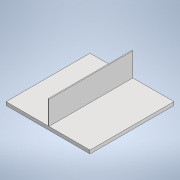
# Autodesk Inventor part: podłoga
Saved by Autodesk Inventor 2022.3 (Build 263350000, 350)
## iProperties
Created: 2023-01-17
Part Number: podłoga
Material: Generic
Document SubType Name: Modeling
Designer: komputer
Density: 1 g/cm^3
Appearance: Default
Author: komputer
Autodesk Inventor part; units mm, degrees
ref_plane "YZ Plane" through (0, 0, 0) normal (1, 0, 0) x (0, 1, 0)
ref_plane "XZ Plane" through (0, 0, 0) normal (0, 1, 0) x (-1, 0, 0)
ref_plane "XY Plane" through (0, 0, 0) normal (0, 0, 1) x (1, 0, 0)
sketch "Sketch1" plane through (0, 0, 0) normal (0, 1, 0) x (-1, 0, 0)
  line L0 (0, 0) -> (-25, 0)
  line L1 (-25, 0) -> (-25, -25)
  line L2 (-25, -25) -> (0, -25)
  line L3 (0, -25) -> (0, 0)
  line L4 (-12.5, 0) -> (-12.5, -25)
  line L5 (-12.5, 0) -> (-12.772, 0)
  line L6 (-12.772, 0) -> (-12.772, -25)
  line L7 (-25, -25) -> (0, -25)
  line L8 (0, -25) -> (0, -26.7912)
  line L9 (0, -26.7912) -> (-25, -26.7912)
  line L10 (-25, -26.7912) -> (-25, -25)
  line L11 (-12.5, -26.7912) -> (-12.5, -25)
  line L12 (-12.228, 0) -> (-12.228, -25)
  dimension "d0" = 25
  dimension "d1" = 25
  dimension "d2" = 0.272
  constraints: 26 end point, 4 parallel, 4 perpendicular, 3 midpoint, 2 horizontal, 2 point on line, 2 symmetric about line
  measures "d0" distance of L2.end L1.end
  measures "d1" distance of L1.end L0.end
  measures "d2" distance of L4.start L5.end
extrude "Extrusion1" add sketch "Sketch1" against normal blind 3 contours L3 L2 L12 L0 | L12 L2 L4 L0 | L4 L2 L6 L0 | L6 L2 L1 L0
extrude "Extrusion2" add sketch "Sketch1" along normal blind 7 contours L4 L2 L6 L0
extrude "Extrusion3" add sketch "Sketch1" along normal blind 3 contours L12 L2 L4 L0
sketch "Sketch2" plane through (25, -3, -25) normal (0, 0, -1) x (-1, 0, 0)
  line L0 (12.5, 6) -> (12.5, 10) projected
  line L1 (12.5, 10) -> (12.5, 30.188)
  point P0 (25, 3)
  constraints: 2 end point, 1 vertical
body "Solid1"
